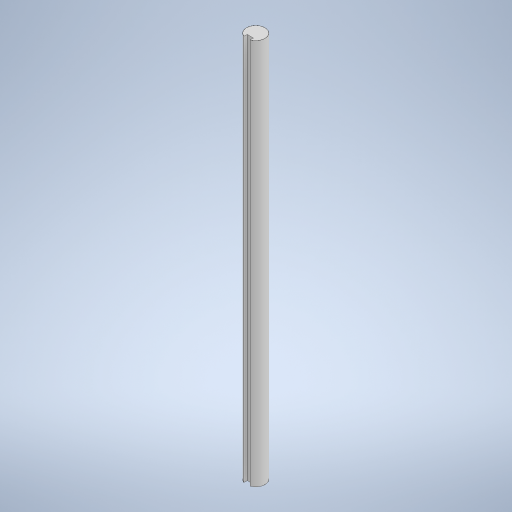
# Autodesk Inventor part: 射出機構_軸2
Saved by Autodesk Inventor 2023 (Build 270158000, 158)
## iProperties
Created: 2022-05-09
Part Number: 射出機構_軸2
Material: 一般
Document SubType Name: Modeling
Designer: yuta
Density: 1 g/cm^3
Appearance: 既定
Author: yuta
Autodesk Inventor part; units mm, degrees
ref_plane "YZ Plane" through (0, 0, 0) normal (1, 0, 0) x (0, 1, 0)
ref_plane "XZ Plane" through (0, 0, 0) normal (0, 1, 0) x (-1, 0, 0)
ref_plane "XY Plane" through (0, 0, 0) normal (0, 0, 1) x (1, 0, 0)
sketch "スケッチ1" plane through (0, 0, 0) normal (0, 1, 0) x (-1, 0, 0)
  circle A0 centre (0, 0) radius 6
  dimension "d0" = 12
  constraints: 1 centre point, 1 coincident
  measures "d0" diameter of A0
extrude "押し出し1" add sketch "スケッチ1" along normal blind 250
sketch "スケッチ2" plane through (0, 250, 0) normal (0, 1, 0) x (1, 0, 0)
  circle A0 centre (0, 0) radius 6 projected
  line L0 (0, -3.5) -> (2, -3.5)
  line L1 (2, -3.5) -> (2, -5.6569)
  circle A1 centre (0, 0) radius 6 projected
  line L2 (0, -3.5) -> (-2, -3.5)
  line L3 (-2, -3.5) -> (-2, -5.6569)
  arc A2 (-2, -5.6569) -> (2, -5.6569) centre (0, 0) ccw
  dimension "d3" = 3.5
  dimension "d4" = 2
  dimension "d5" = 2
  constraints: 8 end point, 4 point on circle, 2 perpendicular, 1 centre point, 1 concentric, 1 horizontal, 1 point on line
  measures "d3" distance of A0.centre L0.start
  measures "d4" distance of L0.start L0.end
  measures "d5" distance of L0.start L2.end
extrude "押し出し2" cut sketch "スケッチ2" against normal blind 250 contours L3 L2 L0 L1 A0 picked at (-0.8927, -4.3205)
